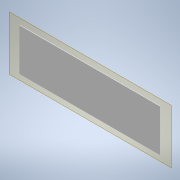
# Autodesk Inventor part: aluminium
Saved by Autodesk Inventor 2021 (Build 250183000, 183)
## iProperties
Created: 2022-01-22
Part Number: aluminium
Material: Generic
Document SubType Name: Modeling
Designer: avan411
Density: 1 g/cm^3
Appearance: Default
Author: avan411
Autodesk Inventor part; units mm, degrees
ref_plane "YZ Plane" through (0, 0, 0) normal (1, 0, 0) x (0, 1, 0)
ref_plane "XZ Plane" through (0, 0, 0) normal (0, 1, 0) x (-1, 0, 0)
ref_plane "XY Plane" through (0, 0, 0) normal (0, 0, 1) x (1, 0, 0)
ref_plane "Work Plane1" through (0, 0, 0) normal (0, 0, 1) x (1, 0, 0)
sketch "Sketch1" plane through (0, 0, 0) normal (0, 0, 1) x (1, 0, 0)
  line L0 (525, 175) -> (-525, 175) projected
  line L1 (525, -175) -> (525, 175) projected
  line L2 (525, -175) -> (525, 175) projected
  line L3 (-525, -175) -> (525, -175) projected
  line L4 (525, -175) -> (525, 175) projected
  line L5 (525, 175) -> (-525, 175) projected
  line L6 (-525, 175) -> (-525, -175) projected
  line L7 (500, -150) -> (-500, -150) projected
  line L8 (-500, -150) -> (-500, 150) projected
  line L9 (-500, 150) -> (500, 150) projected
  line L10 (500, 150) -> (500, -150) projected
  circle A0 centre (0, 165) radius 3 projected
  circle A1 centre (-515, 165) radius 3 projected
  circle A2 centre (515, 165) radius 3 projected
  circle A3 centre (257.5, 165) radius 3 projected
  circle A4 centre (0, -165) radius 3 projected
  circle A5 centre (257.5, -165) radius 3 projected
  circle A6 centre (515, -165) radius 3 projected
  circle A7 centre (-257.5, -165) radius 3 projected
  circle A8 centre (-515, -165) radius 3 projected
  circle A9 centre (-257.5, 165) radius 3 projected
  point P0 (0, 0)
extrude "Extrusion1" add sketch "Sketch1" along normal blind 4 contours L7 L8 L9 L10
body "Solid1"
